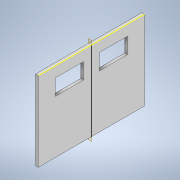
# Autodesk Inventor part: LCD PANEL
Saved by Autodesk Inventor 2020 (Build 240168000, 168)
## iProperties
Created: 2020-04-01
Part Number: LCD PANEL
Material: Generic
Document SubType Name: Modeling
Designer: Yusuf
Density: 1 g/cm^3
Appearance: Default
Author: Yusuf
Autodesk Inventor part; units mm, degrees
ref_plane "YZ Plane" through (0, 0, 0) normal (1, 0, 0) x (0, 1, 0)
ref_plane "XZ Plane" through (0, 0, 0) normal (0, 1, 0) x (-1, 0, 0)
ref_plane "XY Plane" through (0, 0, 0) normal (0, 0, 1) x (1, 0, 0)
sketch "Sketch1" plane through (0, 0, 0) normal (0, 1, 0) x (-1, 0, 0)
  line L0 (-25, 1000) -> (25, 1000)
  line L1 (25, 1000) -> (25, -1000)
  line L2 (25, -1000) -> (-25, -1000)
  line L3 (-25, -1000) -> (-25, 1000)
  line L4 (-25, 1000) -> (25, -1000) construction
  line L5 (25, 1000) -> (-25, -1000) construction
  point P0 (0, 0)
  dimension "d0" = 50
  dimension "d1" = 2000
  constraints: 12 end point, 2 midpoint, 2 parallel, 1 horizontal, 1 perpendicular
  measures "d0" distance of L1.end L2.end
  measures "d1" distance of L0.end L1.end
extrude "Extrusion1" add sketch "Sketch1" along normal blind 1500
sketch "Sketch2" plane through (25, 0, 1000) normal (1, 0, 0) x (0, 0, -1)
  line L0 (2000, 1500) -> (0, 1500) projected
  line L1 (1000, 1500) -> (1000, 0)
  constraints: 2 end point, 1 midpoint, 1 vertical
sketch "Sketch3" plane through (25, 0, 1000) normal (1, 0, 0) x (0, 0, -1)
  line L0 (1150, 1300) -> (1680, 1300)
  line L1 (1680, 1300) -> (1680, 1000)
  line L2 (1680, 1000) -> (1150, 1000)
  line L3 (1150, 1000) -> (1150, 1300)
  line L4 (2000, 0) -> (2000, 1500) projected
  line L5 (1000, 1500) -> (1000, 0) projected
  line L6 (0, 0) -> (2000, 0) projected
  dimension "d4" = 530
  dimension "d5" = 300
  dimension "d6" = 320
  dimension "d7" = 150
  dimension "d8" = 1000
  constraints: 8 end point, 2 parallel, 1 horizontal, 1 perpendicular
  measures "d4" distance of L1.end L2.end
  measures "d5" distance of L0.end L1.end
  measures "d6" distance between parallel lines of L4 L1
  measures "d7" distance between parallel lines of L5 L3
  measures "d8" distance between parallel lines of L6 L2
extrude "Extrusion2" cut sketch "Sketch3" against normal through all
ref_plane "Work Plane1" through (-25, 0, 0) normal (0, 0, 1) x (1, 0, 0)
mirror "Mirror1" about plane through (-25, 0, 0) normal (0, 0, 1) of "Extrusion2"
body "Solid1"
